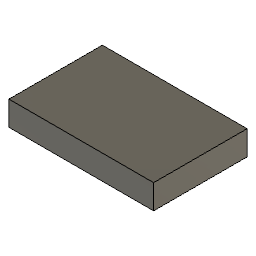
Case_Alex_Mark_Stan (Autodesk Fusion 360 archive; units mm, degrees)
design "LP502030"
part number: 2026-04-10-11-34-23-250
Autodesk Fusion 360 part; units mm, degrees
box "BoxPrimitive1" add length 21 width 32.5 height 5.5 placed x (0, 1, 0) y (-1, 0, 0) z (0, 0, 1) at (0, 0, 0)

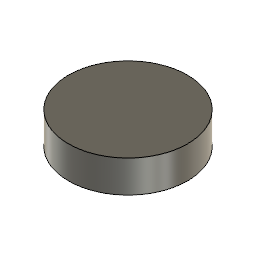
design "FIT0774"
part number: 2026-04-10-12-45-08-588
Autodesk Fusion 360 part; units mm, degrees
cylinder "CylinderPrimitive1" add diameter 10 height 2.7 placed x (1, 0, 0) y (0, 1, 0) z (0, 0, 1) at (-11.9402, 0.2297, 0)
move_body "Move1" bodies 1 to x (1, 0, 0) y (0, 1, 0) z (0, 0, 1) at (12, 0, 0)

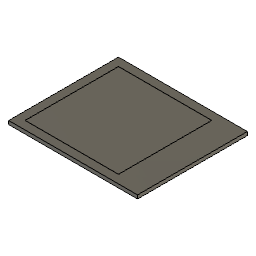
design "15IEPV2"
part number: 2026-04-10-12-06-13-381
Autodesk Fusion 360 part; units mm, degrees
box "BoxPrimitive1" add length 31.8 width 37.32 height 1.05 placed x (0, 1, 0) y (-1, 0, 0) z (0, 0, 1) at (34.32, -1, 0) makes body 1
sketch "Sketch2" plane through (0, 0, 1.05) normal (0, 0, 1) x (-1, 0, 0)
  line L0 (-34.32, -30.8) -> (3, -30.8)
  line L1 (3, -30.8) -> (3, 1)
  line L2 (3, 1) -> (-34.32, 1)
  line L3 (-34.32, 1) -> (-34.32, -30.8)
  line L4 (-26.3996, -1.4003) -> (0.6, -1.4003)
  line L5 (0.6, -1.4003) -> (0.6, -28.4)
  line L6 (0.6, -28.4) -> (-26.3996, -28.4)
  line L7 (-26.3996, -28.4) -> (-26.3996, -1.4003)
  constraint horizontal L4
  constraint vertical L5
  constraint horizontal L6
  constraint vertical L7
surface "SurfacePatch1" add patch profiles "Sketch2" section 1 contours L4 L5 L6 L7 separate body makes body 2
surface "Extrude1" add extruded along (0, 0, 1) between 0 and 0.01 1 faces at (17.3998, 10.4002, 1.05) separate body on bodies 2 makes body 3
named bodies: "Display Area"
